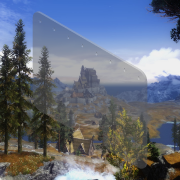
# Autodesk Inventor part: C12_TK_UpperFrameSupport
Saved by Autodesk Inventor 2015 SP1 (Build 190203100, 203)
## iProperties
Created: 2016-01-16
Part Number: C12_TK_UpperFrameSupport
Material: Polycarbonate, Clear
Document SubType Name: Modeling
Designer: TheeTimatahee
Density: 1.2 g/cm^3
Appearance: Polycarbonate - Clear
Mass: 110.596 g
Surface Area: 609.551 cm^2
Volume: 92.1634 cm^3
Author: TheeTimatahee
Autodesk Inventor part; units mm, degrees
ref_plane "YZ Plane" through (0, 0, 0) normal (1, 0, 0) x (0, 1, 0)
ref_plane "XZ Plane" through (0, 0, 0) normal (0, 1, 0) x (-1, 0, 0)
ref_plane "XY Plane" through (0, 0, 0) normal (0, 0, 1) x (1, 0, 0)
sketch "Sketch1" plane through (0, 0, 0) normal (0, 0, 1) x (1, 0, 0)
  line L0 (-101.6, -76.2) -> (101.6, -76.2)
  line L1 (101.6, -76.2) -> (101.6, 76.2)
  line L2 (101.6, 76.2) -> (-101.6, 76.2)
  line L3 (-101.6, 76.2) -> (-101.6, -76.2)
  line L4 (-101.6, -76.2) -> (101.6, 76.2) construction
  line L5 (101.6, -76.2) -> (-101.6, 76.2) construction
  point P0 (0, 0)
  dimension "d0" = 152.4
  dimension "d1" = 203.2
  constraints: 12 end point, 2 midpoint, 2 parallel, 1 horizontal, 1 perpendicular
  measures "d0" distance of L0.end L1.end
  measures "d1" distance of L1.end L2.end
extrude "Extrusion1" add sketch "Sketch1" along normal blind 3.175
fillet "Fillet1" radius 12.7 4 edges at (101.6, 76.2, 1.5875) (101.6, -76.2, 1.5875) (-101.6, -76.2, 1.5875) (-101.6, 76.2, 1.5875)
sketch "Sketch2" plane through (0, 0, 3.175) normal (0, 0, 1) x (1, 0, 0)
  line L0 (101.6, -73.1012) -> (-101.6, -73.1012) projected
  line L1 (101.6, -73.1012) -> (101.6, -53.8988) projected
  line L2 (-101.6, -53.8988) -> (101.6, -53.8988) projected
  line L3 (-97.2058, -18.9992) -> (-97.2058, 44.2468) projected
  line L4 (-97.2058, -18.9992) -> (-85.1719, -18.9992) projected
  line L5 (-85.1719, -18.9992) -> (-31.877, 34.2957) projected
  line L6 (-31.877, 34.2957) -> (-31.877, 46.3296) projected
  line L7 (-95.123, 46.3296) -> (-31.877, 46.3296) projected
  line L8 (-101.6, 63.5) -> (-101.6, -63.5) projected
  line L9 (-88.9, -76.2) -> (88.9, -76.2) projected
  arc A0 (-97.2058, 44.2468) -> (-95.123, 46.3296) centre (-97.1931, 46.3169) ccw projected
  circle A1 centre (-74.2399, 4.9487) radius 2.0701 projected
  circle A2 centre (-56.2794, 41.3242) radius 2.4892 projected
  circle A3 centre (-92.2004, 5.4032) radius 2.4892 projected
  circle A4 centre (-74.2399, 23.3637) radius 14.2875 projected
  circle A5 centre (-74.2399, 41.7787) radius 2.0701 projected
  circle A6 centre (-91.7406, 40.8644) radius 3.7211 projected
  circle A7 centre (-55.8249, 23.3637) radius 2.0701 projected
  circle A8 centre (-92.6549, 23.3637) radius 2.0701 projected
  circle A9 centre (-88.9, -63.5) radius 2.0701 projected
  circle A10 centre (-63.5, -63.5) radius 2.0701 projected
  circle A11 centre (-38.1, -63.5) radius 2.0701 projected
  circle A12 centre (-12.7, -63.5) radius 2.0701 projected
  circle A13 centre (12.7, -63.5) radius 2.0701 projected
  circle A14 centre (38.1, -63.5) radius 2.0701 projected
  circle A15 centre (63.5, -63.5) radius 2.0701 projected
  circle A16 centre (88.9, -63.5) radius 2.0701 projected
  arc A17 (65.5687, 63.5) -> (61.4313, 63.5) centre (63.5, 63.4238) ccw projected
  line L10 (61.4313, 63.5) -> (40.1687, 63.5) projected
  arc A18 (40.1687, 63.5) -> (36.0313, 63.5) centre (38.1, 63.4238) ccw projected
  line L11 (36.0313, 63.5) -> (14.7687, 63.5) projected
  arc A19 (14.7687, 63.5) -> (10.6313, 63.5) centre (12.7, 63.4238) ccw projected
  line L12 (10.6313, 63.5) -> (-10.6313, 63.5) projected
  arc A20 (-10.6313, 63.5) -> (-14.7687, 63.5) centre (-12.7, 63.4238) ccw projected
  line L13 (-14.7687, 63.5) -> (-36.0313, 63.5) projected
  arc A21 (-36.0313, 63.5) -> (-40.1687, 63.5) centre (-38.1, 63.4238) ccw projected
  line L14 (-40.1687, 63.5) -> (-61.4313, 63.5) projected
  arc A22 (-61.4313, 63.5) -> (-65.5687, 63.5) centre (-63.5, 63.4238) ccw projected
  line L15 (-65.5687, 63.5) -> (-86.8313, 63.5) projected
  arc A23 (-86.8313, 63.5) -> (-90.9687, 63.5) centre (-88.9, 63.4238) ccw projected
  line L16 (-90.9687, 63.5) -> (-101.6, 63.5) projected
  line L17 (-101.6, 76.1238) -> (-101.6, 63.5) projected
  line L18 (-101.6, 76.1238) -> (101.6, 76.1238) projected
  line L19 (101.6, 63.5) -> (101.6, 76.1238) projected
  line L20 (101.6, 63.5) -> (90.9687, 63.5) projected
  arc A24 (90.9687, 63.5) -> (86.8313, 63.5) centre (88.9, 63.4238) ccw projected
  line L21 (86.8313, 63.5) -> (65.5687, 63.5) projected
  line L22 (-101.6, -53.8988) -> (-101.6, -73.1012) projected
  point P0 (0, 0)
  point P1 (-88.9, -63.5)
  point P2 (-63.5, -63.5)
  point P3 (-38.1, -63.5)
  point P4 (-12.7, -63.5)
  point P5 (12.7, -63.5)
  point P6 (38.1, -63.5)
  point P7 (63.5, -63.5)
  point P8 (88.9, -63.5)
  dimension "d12" = 12.7
  dimension "d13" = 12.7
  dimension "d16" = 25.4
  constraints: 8 coincident, 1 horizontal, 7 other
  measures "d12" distance from line of L8 point (-88.9, -63.5)
  measures "d13" distance from line of L9 point (-88.9, -63.5)
  measures "d16" distance of point (-88.9, -63.5) point (-63.5, -63.5)
hole "Hole1" at (-63.5, -63.5, 3.175) at (-88.9, -63.5, 3.175) at (-38.1, -63.5, 3.175) at (-12.7, -63.5, 3.175) at (12.7, -63.5, 3.175) at (38.1, -63.5, 3.175) at (63.5, -63.5, 3.175) at (88.9, -63.5, 3.175) at (-88.9, 63.4238, 3.175) at (-63.5, 63.4238, 3.175) at (-38.1, 63.4238, 3.175) at (-12.7, 63.4238, 3.175) at (12.7, 63.4238, 3.175) at (38.1, 63.4238, 3.175) at (63.5, 63.4238, 3.175) at (88.9, 63.4238, 3.175) direction (0, 0, -1) diameter 4.1402 end through all
sketch "Sketch3" plane through (0, 0, 0) normal (0, 0, -1) x (-1, 0, 0)
  line L0 (88.9, -76.2) -> (-88.9, -76.2) projected
  line L1 (25.4, -76.2) -> (-25.4, -76.2)
  line L2 (-25.4, -76.2) -> (-25.4, -44.45)
  line L3 (-25.4, -44.45) -> (25.4, -44.45)
  line L4 (25.4, -44.45) -> (25.4, -76.2)
  line L5 (101.6, 63.5) -> (101.6, -63.5) projected
  point P0 (0, 0)
  dimension "d21" = 50.8
  dimension "d22" = 31.75
  dimension "d23" = 76.2
  constraints: 8 end point, 2 parallel, 1 horizontal, 1 perpendicular, 1 point on line
  measures "d21" distance of L2.end L3.end
  measures "d22" distance of L3.end L1.start
  measures "d23" distance between parallel lines of L5 L4
extrude "Extrusion2" cut sketch "Sketch3" against normal through all
fillet "Fillet2" radius 12.7 4 edges at (-25.4, -76.2, 1.5875) (-25.4, -44.45, 1.5875) (25.4, -44.45, 1.5875) (25.4, -76.2, 1.5875)
body "Solid1"
